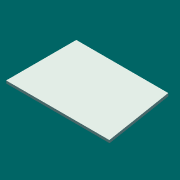
# Autodesk Inventor part: mirrorSides
Saved by Autodesk Inventor 2016 (Build 200138000, 138)
## iProperties
Created: 2015-10-14
Part Number: mirrorSides
Material: Glass
Document SubType Name: Modeling
Designer: Sawaiz
Density: 2.18 g/cm^3
Appearance: Clear
Author: Sawaiz
Autodesk Inventor part; units mm, degrees
ref_plane "XZ Plane" through (0, 0, 0) normal (0, 1, 0) x (-1, 0, 0)
ref_plane "XY Plane" through (0, 0, 0) normal (0, 0, 1) x (1, 0, 0)
sketch "Sketch5" plane through (0, 0, 0) normal (1, 0, 0) x (0, 1, 0)
  line L0 (-60.325, -60.325) -> (60.325, -60.325)
  line L1 (60.325, -60.325) -> (60.325, 60.325)
  line L2 (60.325, 60.325) -> (-60.325, 60.325)
  line L3 (-60.325, 60.325) -> (-60.325, -60.325)
  line L4 (-60.325, -60.325) -> (60.325, 60.325) construction
  line L5 (60.325, -60.325) -> (-60.325, 60.325) construction
  line L6 (-57.15, -57.15) -> (57.15, -57.15)
  line L7 (57.15, -57.15) -> (57.15, 57.15)
  line L8 (57.15, 57.15) -> (-57.15, 57.15)
  line L9 (-57.15, 57.15) -> (-57.15, -57.15)
  line L10 (-57.15, -57.15) -> (57.15, 57.15) construction
  line L11 (57.15, -57.15) -> (-57.15, 57.15) construction
  point P0 (0, 0)
  dimension "d15" = 120.65
  dimension "d16" = 120.65
  dimension "d17" = 114.3
  dimension "d18" = 114.3
  constraints: 24 end point, 4 midpoint, 4 parallel, 2 horizontal, 2 perpendicular
  measures "d15" distance of L2.end L1.end
  measures "d16" distance of L1.end L0.end
  measures "d17" distance of L8.end L7.end
  measures "d18" distance of L7.end L6.end
ref_plane "Work Plane1" through (-71.4375, 0, 0) normal (1, 0, 0) x (0, 1, 0)
sketch "Sketch16" plane through (0, 0, 0) normal (0, 1, 0) x (-1, 0, 0)
  line L0 (0, 57.15) -> (71.4375, 50.9)
  line L1 (71.4375, 50.9) -> (71.4375, 57.15)
  line L2 (71.4375, 57.15) -> (0, 57.15)
  point P0 (0, 0)
  point P1 (0, 57.15)
  dimension "d41" = 5
  dimension "d42" = 71.4375
  constraints: 6 end point, 2 coincident, 1 perpendicular, 1 vertical
  measures "d41" angle of L0 L2
  measures "d42" distance from line of L0.start L1
sketch "Sketch17" plane through (-71.4375, 0, 0) normal (1, 0, 0) x (0, 1, 0)
  line L0 (-50.9, -50.9) -> (50.9, -50.9)
  line L1 (50.9, -50.9) -> (50.9, 50.9)
  line L2 (50.9, 50.9) -> (-50.9, 50.9)
  line L3 (-50.9, 50.9) -> (-50.9, -50.9)
  line L4 (-50.9, -50.9) -> (50.9, 50.9) construction
  line L5 (50.9, -50.9) -> (-50.9, 50.9) construction
  line L6 (-54.075, 54.075) -> (54.075, 54.075)
  line L7 (54.075, 54.075) -> (54.075, -54.075)
  line L8 (54.075, -54.075) -> (-54.075, -54.075)
  line L9 (-54.075, -54.075) -> (-54.075, 54.075)
  point P0 (0, 0)
  point P1 (0, 50.9)
  dimension "d44" = 3.175
  constraints: 20 end point, 4 parallel, 3 midpoint, 3 perpendicular, 1 horizontal, 3 other
  measures "d44" distance between parallel lines of L2 L6
loft "Loft3" add profiles "Sketch5", "Sketch17" contours L3 L2 L1 L0 | L9 L8 L7 L6 / L3 L2 L1 L0 | L6 L7 L8 L9
sketch "Sketch18" plane through (0, -60.325, -60.325) normal (1, 0, 0) x (0, 0, -1)
  line L0 (0, 0) -> (0, 120.65) projected
  line L1 (0, 120.65) -> (-120.65, 120.65) projected
  line L2 (-120.65, 120.65) -> (-120.65, 0) projected
  line L3 (-120.65, 0) -> (0, 0) projected
  line L4 (-117.475, 3.175) -> (-117.475, 117.475)
  line L5 (-117.475, 117.475) -> (-3.175, 117.475)
  line L6 (-3.175, 117.475) -> (-3.175, 3.175)
  line L7 (-3.175, 3.175) -> (-117.475, 3.175)
  point P0 (-60.325, 60.325)
  dimension "d49" = 3.175
  constraints: 8 end point, 3 other
  measures "d49" distance between parallel lines of L2 L4
sketch "Sketch19" plane through (-71.4375, -54.075, -54.075) normal (-1, 0, 0) x (0, 0, 1)
  line L0 (0, 0) -> (0, 108.1501) projected
  line L1 (108.1501, 0) -> (0, 0) projected
  line L2 (108.1501, 108.1501) -> (108.1501, 0) projected
  line L3 (0, 108.1501) -> (108.1501, 108.1501) projected
  line L4 (104.9751, 3.175) -> (3.175, 3.175)
  line L5 (3.175, 3.175) -> (3.175, 104.9751)
  line L6 (3.175, 104.9751) -> (104.9751, 104.9751)
  line L7 (104.9751, 104.9751) -> (104.9751, 3.175)
  point P0 (54.075, 54.075)
  dimension "d50" = 3.175
  constraints: 8 end point, 3 other
  measures "d50" distance between parallel lines of L2 L7
loft "Loft4" cut profiles "Sketch19", "Sketch18" contours L4 L5 L6 L7 / L4 L5 L6 L7
sketch "Sketch20" plane through (0, -57.15, -57.15) normal (0.0871557, 0, 0.9961947) x (0.9961947, 0, -0.0871557)
  line L0 (-71.7104, 6.25) -> (-71.7104, 108.05) projected
  line L1 (-71.7104, 6.25) -> (0, 0) projected
  line L2 (0, 114.3) -> (0, 0) projected
  line L3 (-71.7104, 108.05) -> (0, 114.3) projected
  point P0 (-4.981, 57.15)
extrude "Extrusion6" cut sketch "Sketch20" against normal through all keep common part
equation "\"d15\" = width - internalAcrylicThickness"
equation "\"d16\" = height - internalAcrylicThicnkess"
equation "\"d17\" = -2 * mirrorThickness + width - internalAcrylicThickness"
equation "\"d18\" = -internalAcrylicThicnkess + height - 2 * mirrorThickness"
equation "\"d41\" = mirrorAngle"
equation "\"d44\" = mirrorThickness"
equation "\"d49\" = mirrorThickness"
equation "\"d50\" = mirrorThickness"
equation "\"width\" = 127"
equation "\"depth\" = 146.05"
equation "\"mirrorAngle\" = 5deg"
equation "\"mirrorThickness\" = 3.175"
equation "\"fresnelThickness\" = 0.1"
equation "\"centerThickness\" = 1.524"
equation "\"acrylicThickness\" = 6.35"
equation "\"height\" = 127"
equation "\"detectorWidth\" = 52"
equation "\"detectorHeight\" = 52"
equation "\"focalLength\" = 76.2"
equation "\"ior\" = 1.49"
equation "\"fresnelAngle\" = 90deg"
equation "\"fresnelEffectiveDiameter\" = 152.4"
equation "\"mirrorSuppourtWidth\" = 38.1"
equation "\"backGrooveBit\" = 4.8006"
equation "\"sensorHolderWidth\" = 88.9"
equation "\"sensorHolderHeight\" = 88.9"
equation "\"sensorHolderSensorHeight\" = 53.975"
equation "\"sensorHolderSensorWidth\" = 53.975"
equation "\"oRingWidth\" = 1.5875"
equation "\"sensorHolderORingID\" = 203.2"
equation "\"sensorHolderFlushORingID\" = 304.8"
equation "\"frontBackORingID\" = 419.1"
equation "\"mirrorGroove\" = 19.05"
equation "\"backMirrorGroove\" = 6.35"
equation "\"fresnelMirrorChamfer\" = 6.35"
equation "\"mirrorGrooveMill\" = 3.175"
equation "\"detectorOpeningWidth\" = 76.2"
equation "\"detectorOpeningHeight\" = 76.2"
equation "\"sensorHolderDepth\" = 19.05"
equation "\"frameAcrylicThickness\" = 9.525"
equation "\"internalAcrylicThicnkess\" = 6.35"
equation "\"internalAcrylicThickness\" = 6.35"
equation "\"aerogelClearence\" = 3.175"
equation "\"backplanePCBHeight\" = 76.2"
equation "\"backplaneHoleOffsett\" = 6.35"
equation "\"backplanePCBWidth\" = 76.2"
equation "\"backplanePostionOffsett\" = 12.7"
equation "\"moduleSlotClearence\" = 0.79375"
equation "\"plasticThickness\" = 6.35"
equation "\"aerogelHolderDepth\" = 37.30625"
body "Solid3"
